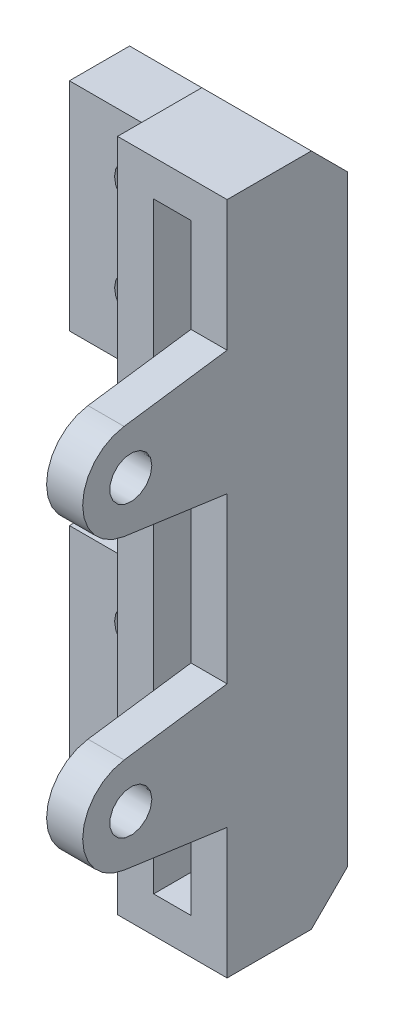
# Autodesk Inventor part: Lysekrone_adapter
Saved by Autodesk Inventor 2023.4 (Build 274418000, 418)
## iProperties
Created: 2025-10-22
Part Number: Lysekrone_adapter
Material: Generic
Document SubType Name: Modeling
Designer: Malthe Sennels
Density: 1 g/cm^3
Appearance: Default
Author: Malthe Sennels
Autodesk Inventor part; units mm, degrees
ref_plane "YZ Plane" through (0, 0, 0) normal (1, 0, 0) x (0, 1, 0)
ref_plane "XZ Plane" through (0, 0, 0) normal (0, 1, 0) x (-1, 0, 0)
ref_plane "XY Plane" through (0, 0, 0) normal (0, 0, 1) x (1, 0, 0)
sketch "Sketch1" plane through (0, 0, 0) normal (0, 0, 1) x (1, 0, 0)
  arc A0 (5.5, 7) -> (3.5, 9) centre (3.5, 7) ccw projected
  line L0 (3.5, 9) -> (-5.5, 9) projected
  line L1 (-5.5, -9) -> (-5.5, 9) projected
  line L2 (-5.5, -9) -> (3.5, -9) projected
  arc A1 (3.5, -9) -> (5.5, -7) centre (3.5, -7) ccw projected
  line L3 (5.5, -7) -> (5.5, 7) projected
  circle A2 centre (0, 4) radius 2.25 construction
  circle A3 centre (0, -4) radius 2.25 construction
  arc A4 (5.5, 39) -> (3.5, 41) centre (3.5, 39) ccw projected
  line L4 (3.5, 41) -> (-5.5, 41) projected
  line L5 (-5.5, 23) -> (-5.5, 41) projected
  line L6 (-5.5, 23) -> (3.5, 23) projected
  arc A5 (3.5, 23) -> (5.5, 25) centre (3.5, 25) ccw projected
  line L7 (5.5, 25) -> (5.5, 39) projected
  circle A6 centre (0, 36) radius 2.25 construction
  circle A7 centre (0, 28) radius 2.25 construction
  circle A8 centre (0, 4) radius 1.75
  circle A9 centre (0, -4) radius 1.75
  circle A10 centre (0, 28) radius 1.75
  circle A11 centre (0, 36) radius 1.75
  line L8 (6.4713, 13.5) -> (-5.5, 13.5) construction
  line L9 (-5.5, 18.5) -> (6.4713, 18.5) construction
  line L10 (6.5, -9) -> (9.6, -9)
  line L11 (9.6, -9) -> (9.6, 41)
  line L12 (9.6, 41) -> (6.5, 41)
  line L13 (6.5, 41) -> (6.5, -9)
  line L14 (-1, 9) -> (-1, 23) construction
  line L15 (-1, 16) -> (6.5, 16) construction
  line L16 (3.5, -12) -> (12.6, -12)
  line L17 (12.6, -12) -> (12.6, 44)
  line L18 (12.6, 44) -> (3.5, 44)
  line L19 (3.5, 44) -> (3.5, -12)
  point P0 (0, 0)
  dimension "d0" = 3.5
  dimension "d1" = 3.5
  dimension "d2" = 3.5
  dimension "d3" = 3.5
  dimension "d4" = 3.1
  dimension "d5" = 50
  dimension "d7" = 3
  constraints: 20 end point, 4 centre point, 4 coincident, 4 midpoint, 4 parallel, 3 perpendicular, 1 horizontal, 1 point on line, 3 other
  measures "d0" diameter of A8
  measures "d1" diameter of A9
  measures "d2" diameter of A10
  measures "d3" diameter of A11
  measures "d4" distance of L11.end L12.end
  measures "d5" distance of L10.start L12.end
  measures "d7" distance between parallel lines of L13 L19
extrude "Extrusion1" add sketch "Sketch1" along normal blind 5
sketch "Sketch2" plane through (0, 0, 5) normal (0, 0, 1) x (1, 0, 0)
  line L0 (12.6, 44) -> (3.5, 44) projected
  line L1 (3.5, -12) -> (12.6, -12) projected
  line L2 (12.6, -12) -> (12.6, 44) projected
  line L3 (12.6, -12) -> (3.5, -12)
  line L4 (3.5, -12) -> (3.5, 44)
  line L5 (3.5, 44) -> (12.6, 44)
  line L6 (12.6, 44) -> (12.6, -12)
  line L7 (6.5, -9) -> (6.5, 41) projected
  line L8 (9.6, -9) -> (6.5, -9) projected
  line L9 (6.5, 41) -> (9.6, 41)
  line L10 (9.6, 41) -> (9.6, -9)
  line L11 (9.6, -9) -> (6.5, -9)
  line L12 (6.5, -9) -> (6.5, 41)
  point P0 (0, 0)
  constraints: 16 end point, 4 parallel, 2 horizontal, 2 perpendicular
extrude "Extrusion2" add sketch "Sketch2" along normal blind 5
sketch "Sketch3" plane through (12.6, -12, 0) normal (1, 0, 0) x (0, 0, -1)
  circle A0 centre (-18, 40) radius 1.75
  arc A1 (-18.5567, 43.9611) -> (-18.5567, 36.0389) centre (-18, 40) ccw
  line L0 (-18.5567, 36.0389) -> (-10, 34.8364)
  line L1 (-10, 0) -> (-10, 56) projected
  line L2 (-18.5567, 43.9611) -> (-10, 45.1636)
  line L3 (-18, 40) -> (-10, 40) construction
  line L4 (-33.1913, 28) -> (0, 28)
  line L5 (0, 0) -> (0, 56) projected
  circle A2 centre (-18, 16) radius 1.75
  arc A3 (-18.5567, 19.9611) -> (-18.5567, 12.0389) centre (-18, 16) ccw
  line L6 (-18.5567, 19.9611) -> (-10, 21.1636)
  line L7 (-18.5567, 12.0389) -> (-10, 10.8364)
  line L8 (-18, 16) -> (-10, 16) construction
  point P0 (0, 12)
  point P1 (-14, 40)
  point P2 (-10, 28)
  point P3 (-10, 28)
  point P4 (-14, 16)
  dimension "d12" = 3.5
  dimension "d13" = 8
  dimension "d14" = 8
  dimension "d15" = 4
  dimension "d16" = 8
  dimension "d17" = 12
  constraints: 14 end point, 8 symmetric about line, 4 centre point, 4 midpoint, 4 point on circle, 4 point on line, 2 coincident, 2 tangent, 1 perpendicular, 2 other
  measures "d12" diameter of A0
  measures "d13" angle of L2 L3
  measures "d14" angle of L3 L0
  measures "d15" radius of A1
  measures "d16" distance from line of A0.centre L1
  measures "d17" vertical distance of point (-14, 40) point (-10, 28)
extrude "Extrusion3" add sketch "Sketch3" against normal up to surface (3 mm away)
sketch "Sketch4" plane through (0, 0, 5) normal (0, 0, 1) x (1, 0, 0)
  point P0 (0, 0)
chamfer "Chamfer1" distance 3 angle 45 2 edges at (8.05, 44, 0) (8.05, -12, 0)
body "Solid1"
